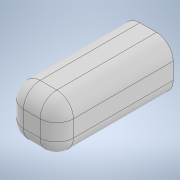
# Autodesk Inventor part: switch cover
Saved by Autodesk Inventor 2020 (Build 240168000, 168)
## iProperties
Created: 2019-06-12
Part Number: switch cover
Material: Generic
Document SubType Name: Modeling
Designer: Holt
Density: 1 g/cm^3
Appearance: Default
Author: Holt
Autodesk Inventor part; units mm, degrees
ref_plane "YZ Plane" through (0, 0, 0) normal (1, 0, 0) x (0, 1, 0)
ref_plane "XZ Plane" through (0, 0, 0) normal (0, 1, 0) x (-1, 0, 0)
ref_plane "XY Plane" through (0, 0, 0) normal (0, 0, 1) x (1, 0, 0)
sketch "Sketch1" plane through (0, 0, 0) normal (0, 0, 1) x (1, 0, 0)
  line L0 (-1, 1) -> (1, 1)
  line L1 (1, 1) -> (1, -1)
  line L2 (1, -1) -> (-1, -1)
  line L3 (-1, -1) -> (-1, 1)
  line L4 (-1, 1) -> (1, -1) construction
  line L5 (1, 1) -> (-1, -1) construction
  line L6 (3, 3) -> (-3, 3)
  line L7 (-3, 3) -> (-3, -3)
  line L8 (-3, -3) -> (3, -3)
  line L9 (3, -3) -> (3, 3)
  point P0 (0, 0)
  dimension "d0" = 2
  dimension "d1" = 2
  dimension "d2" = 2
  constraints: 20 end point, 4 parallel, 2 midpoint, 2 perpendicular, 1 horizontal, 3 other
  measures "d0" distance of L1.end L2.end
  measures "d1" distance of L0.end L1.end
  measures "d2" distance between parallel lines of L0 L6
extrude "Extrusion1" add sketch "Sketch1" along normal blind 14
sketch "Sketch2" plane through (0, 0, 14) normal (0, 0, 1) x (1, 0, 0)
  line L0 (-3, -3) -> (3, -3) projected
  line L1 (3, -3) -> (3, 3) projected
  line L2 (3, 3) -> (-3, 3) projected
  line L3 (-3, 3) -> (-3, -3) projected
  line L4 (1, -1) -> (-1, -1) projected
  line L5 (-1, -1) -> (-1, 1) projected
  line L6 (-1, 1) -> (1, 1) projected
  line L7 (1, 1) -> (1, -1) projected
  point P0 (0, 0)
extrude "Extrusion2" add sketch "Sketch2" against normal blind 8 contours L4 L5 L6 L7
fillet "Fillet1" radius 2 8 edges at (3, 3, 7) (-3, 3, 7) (-3, -3, 7) (3, -3, 7) (3, 0, 14) (0, -3, 14) (-3, 0, 14) (0, 3, 14)
sketch "Sketch3" plane through (0, 0, 0) normal (0, 0, -1) x (-1, 0, 0)
  arc A0 (1, -3) -> (3, -1) centre (1, -1) ccw projected
  line L0 (3, 1) -> (3, -1) projected
  arc A1 (3, 1) -> (1, 3) centre (1, 1) ccw projected
  line L1 (-1, 3) -> (1, 3) projected
  arc A2 (-1, 3) -> (-3, 1) centre (-1, 1) ccw projected
  line L2 (-3, -1) -> (-3, 1) projected
  arc A3 (-3, -1) -> (-1, -3) centre (-1, -1) ccw projected
  line L3 (1, -3) -> (-1, -3) projected
  line L4 (-1, -1) -> (1, -1) projected
  line L5 (-1, 1) -> (-1, -1) projected
  line L6 (1, 1) -> (-1, 1) projected
  line L7 (1, -1) -> (1, 1) projected
  line L8 (-1.25, -1.25) -> (1.25, -1.25)
  line L9 (1.25, -1.25) -> (1.25, 1.25)
  line L10 (1.25, 1.25) -> (-1.25, 1.25)
  line L11 (-1.25, 1.25) -> (-1.25, -1.25)
  point P0 (0, 0)
  dimension "d8" = 0.25
  constraints: 8 end point, 3 other
  measures "d8" distance between parallel lines of L5 L11
extrude "Extrusion3" cut sketch "Sketch3" against normal blind 6 contours L5 L6 L7 L4 | L11 L10 L9 L8
body "Solid1"
